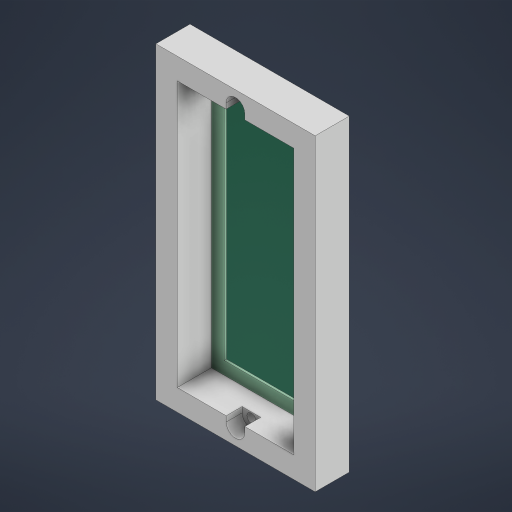
# Autodesk Inventor part: base
Saved by Autodesk Inventor 2024.3 (Build 283343000, 343)
## iProperties
Created: 2025-08-11
Part Number: base
Material: Generic
Document SubType Name: Modeling
Designer: giuseppe
Density: 1 g/cm^3
Appearance: Default
Author: giuseppe
## iProperties of the stored document base_3DPrint.ipt
Created: 2025-08-11
Part Number: base_3DPrint
Material: Generic
Document SubType Name: Modeling
Designer: giuseppe
Density: 1 g/cm^3
Appearance: Default
Author: giuseppe
Autodesk Inventor part; units mm, degrees
ref_plane "YZ Plane" through (0, 0, 0) normal (1, 0, 0) x (0, 1, 0)
ref_plane "XZ Plane" through (0, 0, 0) normal (0, 1, 0) x (-1, 0, 0)
ref_plane "XY Plane" through (0, 0, 0) normal (0, 0, 1) x (1, 0, 0)
ref_plane "Work Plane1" through (0, 0, -3) normal (0, 0, -1) x (-1, 0, 0)
sketch "Sketch1" plane through (0, 0, -3) normal (0, 0, -1) x (-1, 0, 0)
  line L0 (25, 57.75) -> (-25, 57.75) construction
  line L1 (25, -57.75) -> (25, 57.75) construction
  line L2 (-25, 57.75) -> (-25, -57.75) construction
  line L3 (-25, -57.75) -> (25, -57.75) construction
  line L4 (2, -8.6027) -> (2, -14.75) construction
  line L5 (2, -14.75) -> (-17, -5.2524) construction
  line L6 (-17, -5.2524) -> (-2, -7.8973) construction
  line L7 (-2, -7.8973) -> (-2, -1.75) construction
  line L8 (-2, -1.75) -> (17, -11.2476) construction
  line L9 (17, -11.2476) -> (2, -8.6027) construction
  line L10 (2, 40.8973) -> (2, 34.75) construction
  line L11 (2, 34.75) -> (-17, 44.2476) construction
  line L12 (-17, 44.2476) -> (-2, 41.6027) construction
  line L13 (-2, 41.6027) -> (-2, 47.75) construction
  line L14 (-2, 47.75) -> (17, 38.2524) construction
  line L15 (17, 38.2524) -> (2, 40.8973) construction
  line L16 (2, -25.1027) -> (2, -31.25) construction
  line L17 (2, -31.25) -> (-17, -21.7524) construction
  line L18 (-17, -21.7524) -> (-2, -24.3973) construction
  line L19 (-2, -24.3973) -> (-2, -18.25) construction
  line L20 (-2, -18.25) -> (17, -27.7476) construction
  line L21 (17, -27.7476) -> (2, -25.1027) construction
  line L22 (2, 7.8973) -> (2, 1.75) construction
  line L23 (2, 1.75) -> (-17, 11.2476) construction
  line L24 (-17, 11.2476) -> (-2, 8.6027) construction
  line L25 (-2, 8.6027) -> (-2, 14.75) construction
  line L26 (-2, 14.75) -> (17, 5.2524) construction
  line L27 (17, 5.2524) -> (2, 7.8973) construction
  line L28 (2, 24.3973) -> (2, 18.25) construction
  line L29 (2, 18.25) -> (-17, 27.7476) construction
  line L30 (-17, 27.7476) -> (-2, 25.1027) construction
  line L31 (-2, 25.1027) -> (-2, 31.25) construction
  line L32 (-2, 31.25) -> (17, 21.7524) construction
  line L33 (17, 21.7524) -> (2, 24.3973) construction
  line L34 (2, -41.6027) -> (2, -47.75) construction
  line L35 (2, -47.75) -> (-17, -38.2524) construction
  line L36 (-17, -38.2524) -> (-2, -40.8973) construction
  line L37 (-2, -40.8973) -> (-2, -34.75) construction
  line L38 (-2, -34.75) -> (17, -44.2476) construction
  line L39 (17, -44.2476) -> (2, -41.6027) construction
  line L40 (-25, 57.75) -> (-25, -57.75) construction
  line L41 (-25, -57.75) -> (25, -57.75) construction
  line L42 (25, -57.75) -> (25, 57.75) construction
  line L43 (25, 57.75) -> (-25, 57.75) construction
  line L44 (20, 52.75) -> (-20, 52.75)
  line L45 (-20, 52.75) -> (-20, -52.75)
  line L46 (-20, -52.75) -> (20, -52.75)
  line L47 (20, -52.75) -> (20, 52.75)
  line L48 (35, 67.75) -> (-35, 67.75)
  line L49 (-35, 67.75) -> (-35, -67.75)
  line L50 (-35, -67.75) -> (35, -67.75)
  line L51 (35, -67.75) -> (35, 67.75)
  point P0 (0, 0)
  dimension "d0" = 5
  dimension "d1" = 5
  dimension "d2" = 5
  dimension "d3" = 5
  dimension "d4" = 15
  dimension "d5" = 15
  dimension "d6" = 15
  dimension "d7" = 15
  constraints: 16 end point, 4 parallel, 2 horizontal, 2 perpendicular
  measures "d0" distance between parallel lines of L42 L47
  measures "d1" distance between parallel lines of L0 L44
  measures "d2" distance between parallel lines of L2 L45
  measures "d3" distance between parallel lines of L3 L46
  measures "d4" distance between parallel lines of L51 L47
  measures "d5" distance between parallel lines of L48 L44
  measures "d6" distance between parallel lines of L50 L46
  measures "d7" distance between parallel lines of L45 L49
extrude "Extrusion1" add sketch "Sketch1" along normal blind 3
sketch "Sketch2" plane through (0, 0, -3) normal (0, 0, 1) x (1, 0, 0)
  line L0 (-2, -8.6027) -> (-2, -14.75) construction
  line L1 (-2, -14.75) -> (17, -5.2524) construction
  line L2 (17, -5.2524) -> (2, -7.8973) construction
  line L3 (2, -7.8973) -> (2, -1.75) construction
  line L4 (2, -1.75) -> (-17, -11.2476) construction
  line L5 (-17, -11.2476) -> (-2, -8.6027) construction
  line L6 (-2, 40.8973) -> (-2, 34.75) construction
  line L7 (-2, 34.75) -> (17, 44.2476) construction
  line L8 (17, 44.2476) -> (2, 41.6027) construction
  line L9 (2, 41.6027) -> (2, 47.75) construction
  line L10 (2, 47.75) -> (-17, 38.2524) construction
  line L11 (-17, 38.2524) -> (-2, 40.8973) construction
  line L12 (-2, -25.1027) -> (-2, -31.25) construction
  line L13 (-2, -31.25) -> (17, -21.7524) construction
  line L14 (17, -21.7524) -> (2, -24.3973) construction
  line L15 (2, -24.3973) -> (2, -18.25) construction
  line L16 (2, -18.25) -> (-17, -27.7476) construction
  line L17 (-17, -27.7476) -> (-2, -25.1027) construction
  line L18 (-2, 7.8973) -> (-2, 1.75) construction
  line L19 (-2, 1.75) -> (17, 11.2476) construction
  line L20 (17, 11.2476) -> (2, 8.6027) construction
  line L21 (2, 8.6027) -> (2, 14.75) construction
  line L22 (2, 14.75) -> (-17, 5.2524) construction
  line L23 (-17, 5.2524) -> (-2, 7.8973) construction
  line L24 (-2, 24.3973) -> (-2, 18.25) construction
  line L25 (-2, 18.25) -> (17, 27.7476) construction
  line L26 (17, 27.7476) -> (2, 25.1027) construction
  line L27 (2, 25.1027) -> (2, 31.25) construction
  line L28 (2, 31.25) -> (-17, 21.7524) construction
  line L29 (-17, 21.7524) -> (-2, 24.3973) construction
  line L30 (-2, -41.6027) -> (-2, -47.75) construction
  line L31 (-2, -47.75) -> (17, -38.2524) construction
  line L32 (17, -38.2524) -> (2, -40.8973) construction
  line L33 (2, -40.8973) -> (2, -34.75) construction
  line L34 (2, -34.75) -> (-17, -44.2476) construction
  line L35 (-17, -44.2476) -> (-2, -41.6027) construction
  line L36 (25, 57.75) -> (25, -57.75) construction
  line L37 (25, -57.75) -> (-25, -57.75) construction
  line L38 (-25, -57.75) -> (-25, 57.75) construction
  line L39 (-25, 57.75) -> (25, 57.75) construction
  line L40 (-25.6, -58.35) -> (25.6, -58.35)
  line L41 (25.6, -58.35) -> (25.6, 58.35)
  line L42 (25.6, 58.35) -> (-25.6, 58.35)
  line L43 (-25.6, 58.35) -> (-25.6, -58.35)
  line L44 (35, 67.75) -> (35, -67.75) projected
  line L45 (-35, 67.75) -> (35, 67.75) projected
  line L46 (-35, -67.75) -> (-35, 67.75) projected
  line L47 (35, -67.75) -> (-35, -67.75) projected
  line L48 (-20, 52.75) -> (-20, -52.75) projected
  line L49 (20, 52.75) -> (-20, 52.75) projected
  line L50 (20, -52.75) -> (20, 52.75) projected
  line L51 (-20, -52.75) -> (20, -52.75) projected
  point P0 (0, 0)
  dimension "d10" = 0.6
  constraints: 8 end point, 3 other
  measures "d10" distance between parallel lines of L37 L40
extrude "Extrusion2" add sketch "Sketch2" along normal blind 15 contours L44 L47 L46 L45
chamfer "Chamfer1" distance 3 angle 45 4 edges at (0, -67.75, -6) (-35, 0, -6) (35, 0, -6) (0, 67.75, -6)
chamfer "Chamfer2" distance 2 angle 45 4 edges at (0, -52.75, -6) (-20, 0, -6) (20, 0, -6) (0, 52.75, -6)
sketch "Sketch3" plane through (0, 0, 12) normal (0, 0, 1) x (1, 0, 0)
  arc A0 (-25, -48.0971) -> (-25, -42.0971) centre (-25, -45.0971) ccw construction
  line L0 (-25, -48.0971) -> (-25, -57.75) construction
  line L1 (-25, -57.75) -> (-3.5, -57.75) construction
  line L2 (-3.5, -57.75) -> (-3.5, -60.75) construction
  arc A1 (-3.5, -60.75) -> (3.5, -60.75) centre (0, -60.75) ccw construction
  line L3 (3.5, -60.75) -> (3.5, -57.75) construction
  line L4 (3.5, -57.75) -> (25, -57.75) construction
  line L5 (25, -57.75) -> (25, 57.75) construction
  line L6 (25, 57.75) -> (3.5, 57.75) construction
  line L7 (3.5, 60.75) -> (3.5, 57.75) construction
  arc A2 (3.5, 60.75) -> (-3.5, 60.75) centre (0, 60.75) ccw construction
  line L8 (-3.5, 57.75) -> (-3.5, 60.75) construction
  line L9 (-3.5, 57.75) -> (-25, 57.75) construction
  line L10 (-25, 57.75) -> (-25, 48.0971) construction
  arc A3 (-25, 42.0971) -> (-25, 48.0971) centre (-25, 45.0971) ccw construction
  line L11 (-25, 42.0971) -> (-25, -42.0971) construction
  circle A4 centre (0, -60.75) radius 1.65 construction
  circle A5 centre (0, 60.75) radius 1.65 construction
  arc A6 (4.1, 60.75) -> (-4.1, 60.75) centre (0, 60.75) ccw
  line L12 (4.1, 60.75) -> (4.1, 58.35)
  line L13 (4.1, 58.35) -> (25.6, 58.35)
  line L14 (25.6, 58.35) -> (25.6, -58.35)
  line L15 (25.6, -58.35) -> (4.1, -58.35)
  line L16 (4.1, -58.35) -> (4.1, -60.75)
  arc A7 (-4.1, -60.75) -> (4.1, -60.75) centre (0, -60.75) ccw
  line L17 (-4.1, -60.75) -> (-4.1, -58.35)
  line L18 (-4.1, -58.35) -> (-25.6, -58.35)
  line L19 (-25.6, -58.35) -> (-25.6, -47.4209)
  arc A8 (-25.6, -47.4209) -> (-25.6, -42.7733) centre (-25, -45.0971) ccw
  line L20 (-25.6, -42.7733) -> (-25.6, 42.7733)
  arc A9 (-25.6, 42.7733) -> (-25.6, 47.4209) centre (-25, 45.0971) ccw
  line L21 (-25.6, 47.4209) -> (-25.6, 58.35)
  line L22 (-25.6, 58.35) -> (-4.1, 58.35)
  line L23 (-4.1, 58.35) -> (-4.1, 60.75)
  line L24 (-4.1, 58.35) -> (4.1, 58.35)
  point P0 (0, 0)
  dimension "d19" = 0.6
  constraints: 26 end point, 8 point on circle, 4 centre point, 1 perpendicular, 15 other
  measures "d19" radial gap between concentric circles of A2 A6
extrude "Extrusion3" cut sketch "Sketch3" against normal blind 7 contours L12 L24 L23 A6
sketch "Sketch4" plane through (0, 0, 5) normal (0, 0, 1) x (1, 0, 0)
  circle A0 centre (0, 60.75) radius 1.65 projected
  point P0 (0, 0)
hole "Hole1" at (0, 60.75, 5) direction (0, 0, -1) diameter 4 depth 7
mirror "Mirror1" about plane through (0, 0, 0) normal (0, 1, 0) of "Hole1", "Extrusion3"
body "Solid1"
